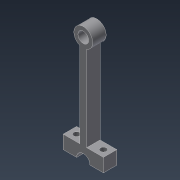
# Autodesk Inventor part: P012-Corps_bielle
Saved by Autodesk Inventor 2021.3 (Build 253353000, 353)
## iProperties
Created: 2022-03-31
Part Number: P012-Corps_bielle
Material: Générique
Document SubType Name: Modeling
Designer: remi
Density: 1 g/cm^3
Appearance: Par défaut
Author: remi
Autodesk Inventor part; units mm, degrees
ref_plane "YZ Plane" through (0, 0, 0) normal (1, 0, 0) x (0, 1, 0)
ref_plane "XZ Plane" through (0, 0, 0) normal (0, 1, 0) x (-1, 0, 0)
ref_plane "XY Plane" through (0, 0, 0) normal (0, 0, 1) x (1, 0, 0)
sketch "Sketch2" plane through (0, 0, 0) normal (0, 1, 0) x (-1, 0, 0)
  line L0 (0, -17.4) -> (0, 104.4) construction
  circle A0 centre (0, 80) radius 4
  arc A1 (2.5, 73.4617) -> (-2.5, 73.4617) centre (0, 80) ccw
  line L1 (-2.5, 73.4617) -> (-2.5, 10)
  line L2 (-2.5, 10) -> (-15, 10)
  line L3 (-15, 10) -> (-15, 0)
  line L4 (-15, 0) -> (-5, 0)
  arc A2 (5, 0) -> (-5, 0) centre (0, 0) ccw
  line L5 (5, 0) -> (15, 0)
  line L6 (15, 0) -> (15, 10)
  line L7 (15, 10) -> (2.5, 10)
  line L8 (2.5, 10) -> (2.5, 73.4617)
  dimension "d0" = 5
  dimension "d2" = 10
  dimension "d3" = 5
  dimension "d7" = 3
  dimension "d8" = 8
  dimension "d20" = 10
  dimension "d22" = 80
  constraints: 16 end point, 6 perpendicular, 4 equal length, 4 point on circle, 3 centre point, 1 coincident, 1 horizontal, 1 horizontal alignment, 1 point on line, 1 vertical
  measures "d0" distance between parallel lines of L1 L8
  measures "d2" distance of L3.end L4.end
  measures "d3" radius of A2
  measures "d7" radial gap between concentric circles of A0 A1
  measures "d8" diameter of A0
  measures "d20" distance from line of A2.centre L2
  measures "d22" distance of A2.centre A0.centre
extrude "Extrusion1" add sketch "Sketch2" along normal blind 10
sketch "Sketch3" plane through (0, 0, 0) normal (0, 0, 1) x (1, 0, 0)
  line L0 (-5, 0) -> (-15, 0) construction
  line L1 (-15, 0) -> (-15, 10) construction
  line L2 (-5, 10) -> (-15, 10) construction
  line L3 (-5, 0) -> (-5, 10) construction
  line L4 (15, 0) -> (5, 0) construction
  line L5 (5, 0) -> (5, 10) construction
  line L6 (15, 10) -> (5, 10) construction
  line L7 (15, 0) -> (15, 10) construction
  line L8 (-15, 0) -> (-5, 10) construction
  line L9 (-5, 0) -> (-15, 10) construction
  line L10 (5, 0) -> (15, 10) construction
  line L11 (15, 0) -> (5, 10) construction
  point P0 (0, 0)
  point P1 (-10, 5)
  point P2 (10, 5)
  constraints: 8 end point, 3 perpendicular, 2 midpoint
hole "Hole1" at (-10, 5, 0) at (10, 5, 0) direction (0, 0, 1) diameter 4.5 depth 10 clearance for "Flat Head Machine Screw" size "M4" standard "Ansi Metric M Profile"
body "Solid1"
